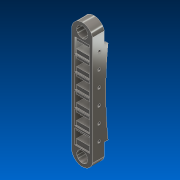
# Autodesk Inventor part: Ponte menor
Saved by Autodesk Inventor 2016 (Build 200138000, 138)
## iProperties
Created: 2018-12-07
Part Number: Ponte menor
Material: Steel
Document SubType Name: Modeling
Designer: lesly
Density: 7.85 g/cm^3
Appearance: Steel - Polished
Author: lesly
Autodesk Inventor part; units mm, degrees
ref_plane "YZ Plane" through (0, 0, 0) normal (1, 0, 0) x (0, 1, 0)
ref_plane "XY Plane" through (0, 0, 0) normal (0, 0, 1) x (1, 0, 0)
sketch "Sketch1" plane through (0, 0, 0) normal (1, 0, 0) x (0, 1, 0)
  line L0 (0, 0) -> (0, -85)
  line L1 (0, -85) -> (8, -85)
  line L2 (0, 0) -> (8, 0)
  line L3 (8, 0) -> (8, -14)
  line L4 (8, -85) -> (8, -71)
  line L5 (8, -14) -> (9, -14)
  line L6 (8, -71) -> (9, -71)
  arc A0 (10.5, -14.5) -> (10.5, -70.5) centre (267.5593, -42.5) ccw
  line L7 (8, -71) -> (10.555, -71)
  line L8 (8, -14) -> (10.555, -14)
  arc A1 (10.555, -14) -> (10.555, -71) centre (267.5473, -42.5) ccw
  constraints: 18 end point, 6 horizontal, 4 point on circle, 3 vertical, 2 centre point
extrude "Extrusion1" add sketch "Sketch1" along normal mid plane 14
sketch "Sketch2" plane through (-7, 8, 0) normal (0, 1, 0) x (1, 0, 0)
  line L0 (0, 85) -> (0, 0) projected
  line L1 (0, 14.0338) -> (0, 5.5338)
  line L2 (14, 0) -> (14, 85) projected
  line L3 (14, 14.0338) -> (14, 5.5338)
  arc A0 (0, 5.5338) -> (14, 5.5338) centre (7, 7.1942) ccw
  line L4 (0, 5.5338) -> (0, 0)
  line L5 (0, 0) -> (14, 0) projected
  line L6 (14, 0) -> (14, 5.5338)
  point P0 (7, 0)
  dimension "d13" = 8.5
  constraints: 8 end point, 4 point on line, 3 point on circle, 1 centre point, 1 collinear, 1 vertical
  measures "d13" distance of L1.start L1.end
extrude "Extrusion2" cut sketch "Sketch2" against normal blind 14
sketch "Sketch3" plane through (-7, 8, -71) normal (0, 1, 0) x (1, 0, 0)
  line L0 (0, 0) -> (14, 0) projected
  line L1 (0, 0) -> (0, 14) projected
  arc A0 (14, 8.5) -> (0, 8.5) centre (7, 6.7955) ccw
  line L2 (0, 8.5) -> (0, 14)
  line L3 (0, 14) -> (14, 14) projected
  line L4 (14, 14) -> (14, 8.5)
  line L5 (14, -65.4662) -> (14, 14) projected
  line L6 (0, 14) -> (0, 8.5)
  line L7 (14, 8.5) -> (14, 14)
  line L8 (14, 14) -> (0, 14)
  line L9 (0, 8.5) -> (0, 14)
  line L10 (0, 14) -> (14, 14) projected
  line L11 (14, 14) -> (14, 8.5)
  line L12 (14, 14) -> (14, 0) projected
  arc A1 (14, 8.5) -> (0, 8.5) centre (7, 6.7955) ccw
  point P0 (7, -71)
  constraints: 14 end point, 5 point on circle, 3 collinear, 2 centre point, 2 point on line, 2 vertical, 1 perpendicular, 1 tangent
extrude "Extrusion3" cut sketch "Sketch3" against normal blind 14 contours L1 L3 A0 | A0 L3 L4
sketch "Sketch7" plane through (0, 0, -7.1942) normal (0, -1, 0) x (1, 0, 0)
  circle A0 centre (0, 2.1942) radius 3 projected
  line L0 (0, -0.8058) -> (0, -3.8058)
  circle A1 centre (0, -72.0142) radius 1.5 projected
  line L1 (0, -70.5142) -> (0, -67.5142)
  line L2 (0, -67.5142) -> (-5, -67.5142)
  line L3 (-5, -67.5142) -> (5, -67.5142)
  line L4 (-5, -67.5142) -> (5, -67.5142)
  line L5 (5, -67.5142) -> (5, -57.4342)
  line L6 (5, -57.4342) -> (-5, -57.4342)
  line L7 (-5, -57.4342) -> (-5, -67.5142)
  line L8 (0, -57.4342) -> (0, -56.9342)
  line L9 (-5, -56.2258) -> (5, -56.2258)
  line L10 (5, -56.2258) -> (5, -46.1458)
  line L11 (5, -46.1458) -> (-5, -46.1458)
  line L12 (-5, -46.1458) -> (-5, -56.2258)
  line L13 (0, -46.1458) -> (0, -45.6458)
  line L14 (-5, -45.6458) -> (5, -45.6458)
  line L15 (5, -45.6458) -> (5, -35.5658)
  line L16 (5, -35.5658) -> (-5, -35.5658)
  line L17 (-5, -35.5658) -> (-5, -45.6458)
  line L18 (0, -35.5658) -> (0, -35.0658)
  line L19 (-5, -35.0658) -> (5, -35.0658)
  line L20 (5, -35.0658) -> (5, -24.9858)
  line L21 (5, -24.9858) -> (-5, -24.9858)
  line L22 (-5, -24.9858) -> (-5, -35.0658)
  line L23 (0, -24.9858) -> (0, -24.4858)
  line L24 (-5, -24.4858) -> (5, -24.4858)
  line L25 (5, -24.4858) -> (5, -14.4058)
  line L26 (5, -14.4058) -> (-5, -14.4058)
  line L27 (-5, -14.4058) -> (-5, -24.4858)
  line L28 (0, -14.4058) -> (0, -13.9058)
  line L29 (-5, -13.9058) -> (5, -13.9058)
  line L30 (5, -13.9058) -> (5, -3.8058)
  line L31 (5, -3.8058) -> (-5, -3.8058)
  line L32 (-5, -3.8058) -> (-5, -13.9058)
  point P0 (0, 7.1942)
  constraints: 66 end point, 12 parallel, 7 horizontal, 6 perpendicular, 6 vertical, 5 midpoint, 2 vertical alignment, 1 point on line, 2 other
extrude "Extrusion6" cut sketch "Sketch7" against normal blind 1 contours L31 L30 L29 L32 | L2 L7 L6 L5 L3
sketch "Sketch8" plane through (0, 0, -7.1942) normal (0, -1, 0) x (1, 0, 0)
  line L0 (-5, -57.4342) -> (5, -57.4342) projected
  line L1 (0, -57.4342) -> (0, -56.9342)
  line L2 (-5, -56.2258) -> (5, -56.2258)
  line L3 (5, -56.2258) -> (5, -46.1458)
  line L4 (5, -46.1458) -> (-5, -46.1458)
  line L5 (-5, -46.1458) -> (-5, -56.2258)
  line L6 (0, -46.1458) -> (0, -45.6458)
  line L7 (-5, -45.6458) -> (5, -45.6458)
  line L8 (5, -45.6458) -> (5, -35.5658)
  line L9 (5, -35.5658) -> (-5, -35.5658)
  line L10 (-5, -35.5658) -> (-5, -45.6458)
  line L11 (0, -35.5658) -> (0, -35.0658)
  line L12 (-5, -35.0658) -> (5, -35.0658)
  line L13 (5, -35.0658) -> (5, -24.9858)
  line L14 (5, -24.9858) -> (-5, -24.9858)
  line L15 (-5, -24.9858) -> (-5, -35.0658)
  line L16 (0, -24.9858) -> (0, -24.4858)
  line L17 (-5, -24.4858) -> (5, -24.4858)
  line L18 (5, -24.4858) -> (5, -14.4058)
  line L19 (5, -14.4058) -> (-5, -14.4058)
  line L20 (-5, -14.4058) -> (-5, -24.4858)
  point P0 (0, 7.1942)
  dimension "d75" = 0.5
  dimension "d76" = 10.08
  dimension "d77" = 0.5
  dimension "d78" = 10.08
  dimension "d79" = 0.5
  dimension "d80" = 10.08
  dimension "d81" = 0.5
  dimension "d82" = 10.08
  constraints: 40 end point, 8 parallel, 4 horizontal, 4 midpoint, 4 perpendicular, 4 vertical, 1 point on line
  measures "d75" distance of L1.start L1.end
  measures "d76" distance of L3.end L2.end
  measures "d77" distance of L6.start L6.end
  measures "d78" distance of L8.end L7.end
  measures "d79" distance of L11.start L11.end
  measures "d80" distance of L13.end L12.end
  measures "d81" distance of L16.start L16.end
  measures "d82" distance of L18.end L17.end
extrude "Extrusion7" cut sketch "Sketch8" against normal blind 1
sketch "Sketch9" plane through (0, 1, -7.1942) normal (0, -1, 0) x (1, 0, 0)
  line L0 (-5, -67.5142) -> (-5, -57.4342) projected
  line L1 (5, -57.4342) -> (5, -67.5142) projected
  line L2 (-5, -59.2658) -> (5, -59.2658)
  line L3 (-5, -64.2658) -> (5, -64.2658)
  line L4 (-5, -64.2658) -> (-5, -59.2658)
  line L5 (5, -64.2658) -> (5, -59.2658)
  line L6 (5, -64.2658) -> (5, -59.2658)
  point P0 (0, 7.1942)
  constraints: 10 end point, 3 collinear
extrude "Extrusion8" cut sketch "Sketch9" against normal blind 20
sketch "Sketch10" plane through (0, 1, -7.1942) normal (0, -1, 0) x (1, 0, 0)
  line L0 (-5, -56.2258) -> (-5, -46.1458) projected
  line L1 (5, -46.1458) -> (5, -56.2258) projected
  line L2 (-5, -53.6858) -> (5, -53.6858)
  line L3 (-5, -48.6858) -> (5, -48.6858)
  line L4 (5, -48.6858) -> (5, -53.6858)
  line L5 (-5, -48.6858) -> (-5, -53.6858)
  point P0 (0, 7.1942)
  dimension "d109" = 5
  constraints: 8 end point, 1 collinear, 1 perpendicular
  measures "d109" distance between parallel lines of L3 L2
extrude "Extrusion9" cut sketch "Sketch10" against normal blind 20
sketch "Sketch11" plane through (0, 1, -7.1942) normal (0, -1, 0) x (1, 0, 0)
  line L0 (-5, -45.6458) -> (-5, -35.5658) projected
  line L1 (5, -35.5658) -> (5, -45.6458) projected
  line L2 (-5, -43.1058) -> (5, -43.1058)
  line L3 (-5, -38.1058) -> (5, -38.1058)
  line L4 (5, -38.1058) -> (5, -43.1058)
  line L5 (-5, -38.1058) -> (-5, -43.1058)
  point P0 (0, 7.1942)
  constraints: 8 end point, 1 parallel, 1 perpendicular
extrude "Extrusion10" cut sketch "Sketch11" against normal blind 20
sketch "Sketch12" plane through (0, 1, -7.1942) normal (0, -1, 0) x (1, 0, 0)
  line L0 (-5, -35.0658) -> (-5, -24.9858) projected
  line L1 (5, -24.9858) -> (5, -35.0658) projected
  line L2 (-5, -32.5258) -> (5, -32.5258)
  line L3 (-5, -27.5258) -> (5, -27.5258)
  line L4 (5, -27.5258) -> (5, -32.5258)
  line L5 (-5, -27.5258) -> (-5, -32.5258)
  point P0 (0, 7.1942)
  constraints: 8 end point, 2 collinear
extrude "Extrusion11" cut sketch "Sketch12" against normal blind 20
sketch "Sketch13" plane through (0, 1, -7.1942) normal (0, -1, 0) x (1, 0, 0)
  line L0 (-5, -24.4858) -> (-5, -14.4058) projected
  line L1 (-5, -21.9458) -> (5, -21.9458)
  line L2 (-5, -16.9458) -> (5, -16.9458)
  line L3 (5, -16.9458) -> (5, -21.9458)
  line L4 (5, -14.4058) -> (5, -24.4858) projected
  line L5 (-5, -16.9458) -> (-5, -21.9458)
  point P0 (0, 7.1942)
  constraints: 8 end point, 2 collinear
extrude "Extrusion12" cut sketch "Sketch13" against normal blind 20
sketch "Sketch14" plane through (0, 1, -7.1942) normal (0, -1, 0) x (1, 0, 0)
  line L0 (-5, -13.9058) -> (-5, -3.8058) projected
  line L1 (5, -3.8058) -> (5, -13.9058) projected
  line L2 (-5, -11.3558) -> (5, -11.3558)
  line L3 (-5, -6.3558) -> (5, -6.3558)
  line L4 (5, -6.3558) -> (5, -11.3558)
  line L5 (-5, -6.772) -> (-5, -11.3558)
  line L6 (-5, -6.3558) -> (-5, -11.3558)
  point P0 (0, 7.1942)
  constraints: 10 end point, 2 collinear, 1 point on line, 1 vertical
extrude "Extrusion13" cut sketch "Sketch14" against normal blind 20
ref_plane "Work Plane1" through (0, 8.9795, -42.5) normal (0, 1, 0) x (-1, 0, 0)
sketch "Sketch30" plane through (0, 0, -7.1942) normal (0, -1, 0) x (1, 0, 0)
  line L0 (7, 1.6605) -> (7, -72.3058) construction
  line L1 (7, -35.3226) -> (-7, -35.3226) construction
  line L2 (-7, -72.3058) -> (-7, 1.6605) construction
  line L3 (0, -35.3226) -> (0, 1.3774) construction
  line L4 (0, -35.3226) -> (0, -72.0226) construction
  circle A0 centre (0, 1.3774) radius 3.75
  circle A1 centre (0, -72.0226) radius 3.75
  point P0 (0, 7.1942)
  dimension "d140" = 36.7
  dimension "d141" = 36.7
  dimension "d142" = 7.5
  dimension "d143" = 7.5
  constraints: 6 end point, 3 midpoint, 2 centre point, 2 coincident, 2 vertical
  measures "d140" distance of L3.start L3.end
  measures "d141" distance of L3.start L4.end
  measures "d142" diameter of A0
  measures "d143" diameter of A1
extrude "Extrusion16" cut sketch "Sketch30" against normal through all
sketch "Sketch31" plane through (7, 0, 0) normal (1, 0, 0) x (0, 0, -1)
  line L0 (13.55, 1) -> (13.55, 8) construction
  line L1 (71.46, 1) -> (71.46, 8) construction
  line L2 (18.55, 1) -> (18.55, 10.0911) construction
  line L3 (24.14, 1) -> (24.14, 9.6322) construction
  line L4 (29.14, 1) -> (29.14, 9.3249) construction
  line L5 (34.72, 1) -> (34.72, 9.0966) construction
  line L6 (39.72, 1) -> (39.72, 8.9945) construction
  line L7 (45.3, 1) -> (45.3, 8.9947) construction
  line L8 (50.3, 1) -> (50.3, 9.0972) construction
  line L9 (55.88, 1) -> (55.88, 9.326) construction
  line L10 (60.88, 1) -> (60.88, 9.6336) construction
  line L11 (66.46, 1) -> (66.46, 10.0921) construction
  line L12 (13.55, 4.5) -> (18.55, 4.5) construction
  line L13 (24.14, 4.5) -> (29.14, 4.5) construction
  line L14 (34.72, 4.5) -> (39.72, 4.5) construction
  line L15 (45.3, 4.5) -> (50.3, 4.5) construction
  line L16 (55.88, 4.5) -> (60.88, 4.5) construction
  line L17 (66.46, 4.5) -> (71.46, 4.5) construction
  circle A0 centre (16.05, 4.5) radius 1
  circle A1 centre (26.64, 4.5) radius 1
  circle A2 centre (37.22, 4.5) radius 1
  circle A3 centre (47.8, 4.5) radius 1
  circle A4 centre (58.38, 4.5) radius 1
  circle A5 centre (68.96, 4.5) radius 1
  point P0 (0, 0)
  dimension "d146" = 2
  dimension "d147" = 2
  dimension "d148" = 2
  dimension "d149" = 2
  dimension "d150" = 2
  dimension "d151" = 2
  constraints: 12 end point, 10 point on line, 8 midpoint, 6 centre point
  measures "d146" diameter of A0
  measures "d147" diameter of A1
  measures "d148" diameter of A2
  measures "d149" diameter of A3
  measures "d150" diameter of A4
  measures "d151" diameter of A5
extrude "Extrusion17" cut sketch "Sketch31" against normal through all
body "Solid1"
